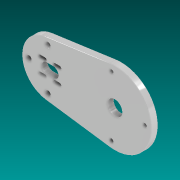
# Autodesk Inventor part: motorplaat
Saved by Autodesk Inventor 2020.2 (Build 242310000, 310)
## iProperties
Created: 2020-05-15
Part Number: motorplaat
Material: Aluminum 6061
Document SubType Name: Modeling
Designer: Svend
Density: 2.7 g/cm^3
Appearance: Aluminum - Polished
Author: Svend
Autodesk Inventor part; units mm, degrees
ref_plane "YZ Plane" through (0, 0, 0) normal (1, 0, 0) x (0, 1, 0)
ref_plane "XZ Plane" through (0, 0, 0) normal (0, 1, 0) x (-1, 0, 0)
ref_plane "XY Plane" through (0, 0, 0) normal (0, 0, 1) x (1, 0, 0)
sketch "Sketch1" plane through (0, 0, 0) normal (0, 0, 1) x (1, 0, 0)
  circle A0 centre (-11.3135, -11.3135) radius 2
  circle A1 centre (-11.3135, 11.3135) radius 2
  circle A2 centre (11.3135, 11.3135) radius 2
  circle A3 centre (11.3135, -11.3135) radius 2
  circle A4 centre (-15.3135, 11.3135) radius 2
  circle A5 centre (-7.3135, 11.3135) radius 2
  circle A6 centre (7.3135, 11.3135) radius 2
  circle A7 centre (15.3135, 11.3135) radius 2
  circle A8 centre (15.3135, -11.3135) radius 2
  circle A9 centre (7.3135, -11.3135) radius 2
  circle A10 centre (-7.3135, -11.3135) radius 2
  circle A11 centre (-15.3135, -11.3135) radius 2
  line L0 (-15.3135, 13.3135) -> (-7.3135, 13.3135)
  line L1 (-7.3135, 9.3135) -> (-15.3135, 9.3135)
  line L2 (-15.3135, -9.3135) -> (-7.3135, -9.3135)
  line L3 (-7.3135, -13.3135) -> (-15.3135, -13.3135)
  line L4 (7.3135, -9.3135) -> (15.3135, -9.3135)
  line L5 (15.3135, -13.3135) -> (7.3135, -13.3135)
  line L6 (15.3135, 9.3135) -> (7.3135, 9.3135)
  line L7 (15.3135, 13.3135) -> (7.3135, 13.3135)
  circle A12 centre (0, 0) radius 8.25
  circle A13 centre (5, 0) radius 8.25
  circle A14 centre (-5, 0) radius 8.25
  line L8 (-5, 8.25) -> (5, 8.25)
  line L9 (5, -8.25) -> (-5, -8.25)
  circle A15 centre (0, 0) radius 42.5
  circle A16 centre (100.143, 0) radius 56.4372
  line L10 (-5.9149, 42.0864) -> (92.2885, 55.888)
  line L11 (-5.9149, -42.0864) -> (92.2885, -55.888)
  line L12 (-13.25, 0) -> (13.25, 0)
  circle A17 centre (100.143, 0) radius 11.5
  arc A18 (-5.9149, 42.0864) -> (-5.9149, -42.0864) centre (0, 0) ccw
  arc A19 (92.2885, -55.888) -> (92.2885, 55.888) centre (100.143, 0) ccw
  line L13 (-42.5, 0) -> (156.5802, 0)
  line L14 (92.2885, 55.888) -> (-5.9149, 42.0864)
  line L15 (-5.9149, -42.0864) -> (92.2885, -55.888)
  line L16 (-3.1314, 22.281) -> (95.0719, 36.0826)
  arc A20 (95.0719, -36.0826) -> (95.0719, 36.0826) centre (100.143, 0) ccw
  line L17 (95.0719, -36.0826) -> (-3.1314, -22.281)
  arc A21 (-3.1314, 22.281) -> (-3.1314, -22.281) centre (0, 0) ccw
  point P0 (146.5802, 0)
  point P1 (95.0719, 46.1809)
  point P2 (95.0719, -46.1809)
  point P3 (-32.5, 0)
  point P4 (-3.1314, 32.3793)
  point P5 (-3.1314, -32.3793)
  dimension "d0" = 4
  dimension "d1" = 22.627
  dimension "d2" = 22.627
  dimension "d3" = 11.3135
  dimension "d4" = 11.3135
  dimension "d5" = 4
  dimension "d6" = 4
  dimension "d7" = 4
  dimension "d8" = 4
  dimension "d9" = 4
  dimension "d10" = 4
  dimension "d11" = 4
  dimension "d12" = 4
  dimension "d15" = 16.5
  dimension "d16" = 5
  dimension "d17" = 5
  dimension "d18" = 85
  dimension "d19" = 8
  dimension "d20" = 100.143
  dimension "d21" = 23
  dimension "d24" = 85
  dimension "d25" = 100.143
  dimension "d26" = 8
  dimension "d27" = 20
  dimension "d28" = 10
  dimension "d29" = 10
  dimension "d30" = 10
  dimension "d31" = 10
  dimension "d32" = 10
  dimension "d33" = 10
  constraints: 36 end point, 36 point on circle, 22 centre point, 15 horizontal alignment, 14 tangent, 13 equal radius, 11 point on line, 6 vertical alignment, 4 coincident, 4 parallel, 3 horizontal, 1 midpoint, 3 other
  measures "d0" diameter of A0
  measures "d1" distance of A1.centre A2.centre
  measures "d2" distance of A3.centre A2.centre
  measures "d3" horizontal distance of point (0, 0) A1.centre
  measures "d4" horizontal distance of point (0, 0) A1.centre
  measures "d5" distance of A2.centre A6.centre
  measures "d6" distance of A7.centre A2.centre
  measures "d7" distance of A3.centre A8.centre
  measures "d8" distance of A9.centre A3.centre
  measures "d9" distance of A0.centre A10.centre
  measures "d10" distance of A11.centre A0.centre
  measures "d11" distance of A1.centre A4.centre
  measures "d12" distance of A5.centre A1.centre
  measures "d15" diameter of A12
  measures "d16" distance of A14.centre A12.centre
  measures "d17" distance of A12.centre A13.centre
  measures "d18" diameter of A15
  measures "d19" angle of L12 L10
  measures "d20" distance of A16.centre point (0, 0)
  measures "d21" diameter of A17
  measures "d24" diameter of A18
  measures "d25" distance of A18.centre A19.centre
  measures "d26" angle of L13 L14
  measures "d27" distance between parallel lines of L14 L16
  measures "d28" distance from line of point (-3.131, -32.379) L17
  measures "d29" distance of L13.end point (146.58, 0)
  measures "d30" distance from line of L16 point (95.072, 46.181)
  measures "d31" distance from line of L16 point (-3.131, 32.379)
  measures "d32" distance from line of point (95.072, -46.181) L17
  measures "d33" distance of L13.start point (-32.5, 0)
extrude "Extrusion1" add sketch "Sketch1" along normal blind 10 contours L13 A15 L17 A21 A14 L9 A13 | A13 L8 A14 L13 A21 L16 A15 | L13 A16 L17 A15 | A15 L16 A16 L13 | L16 A21 L13 A15 | A15 L10 A16 L16 | L17 A16 L11 A15 | A15 L13 A21 L17 | L13 A17 A20 L17 A16 | A16 L16 A20 L13 A17 | A16 L13 A20 L16 | L17 A20 L13 A16
hole "Hole1" at (-3.1314, -32.3793, 0) at (95.0719, -46.1809, 0) at (146.5802, 0, 0) at (95.0719, 46.1809, 0) at (-3.1314, 32.3793, 0) at (-32.5, 0, 0) direction (0, 0, 1) diameter 5.2 depth 10
chamfer "Chamfer1" distance 0.5 angle 45 59 edges at (-42.5, 0, 10) (43.1868, -48.9872, 10) (156.5802, 0, 10) (43.1868, 48.9872, 10) (-42.5, 0, 0) (43.1868, -48.9872, 0) (156.5802, 0, 0) (43.1868, 48.9872, 0) (-5.3135, 11.3135, 10) (-11.3135, 9.3135, 10) (-17.3135, 11.3135, 10) (-11.3135, 13.3135, 10) (-13.25, 0, 10) (0, 8.25, 10) (13.25, 0, 10) (0, -8.25, 10) (-11.3135, -9.3135, 10) (-5.3135, -11.3135, 10) (-11.3135, -13.3135, 10) (-17.3135, -11.3135, 10) (5.3135, 11.3135, 10) (11.3135, 13.3135, 10) (17.3135, 11.3135, 10) (11.3135, 9.3135, 10) (17.3135, -11.3135, 10) (11.3135, -13.3135, 10) (5.3135, -11.3135, 10) (11.3135, -9.3135, 10) (88.643, 0, 0) (88.643, 0, 10) (-5.3135, 11.3135, 0) (-11.3135, 9.3135, 0) (-17.3135, 11.3135, 0) (-11.3135, 13.3135, 0) (-13.25, 0, 0) (0, 8.25, 0) (13.25, 0, 0) (0, -8.25, 0) (-11.3135, -9.3135, 0) (-5.3135, -11.3135, 0) (-11.3135, -13.3135, 0) (-17.3135, -11.3135, 0) (11.3135, 9.3135, 0) (5.3135, 11.3135, 0) (11.3135, 13.3135, 0) (17.3135, 11.3135, 0) (17.3135, -11.3135, 0) (11.3135, -13.3135, 0) (5.3135, -11.3135, 0) (11.3135, -9.3135, 0) (146.5802, -2.6, 0) (95.0719, 43.5809, 0) (95.0719, -48.7809, 0) (-32.5, -2.6, 0) (-3.1314, 29.7793, 0) (-3.1314, -34.9793, 0) (95.0719, -48.7809, 10) (146.5802, -2.6, 10) (95.0719, 43.5809, 10)
chamfer "Chamfer3" distance 2 angle 45 3 edges at (-3.1314, 29.7793, 10) (-32.5, -2.6, 10) (-3.1314, -34.9793, 10)
equation "\"d2\" = d1"
equation "\"d3\" = 0.5 * d2"
equation "\"d4\" = 0.5 * d1"
equation "\"d5\" = d0"
equation "\"d6\" = d5"
equation "\"d7\" = d6"
equation "\"d8\" = d7"
equation "\"d9\" = d5"
equation "\"d10\" = d9"
equation "\"d11\" = d10"
equation "\"d12\" = d11"
equation "\"d17\" = d16"
equation "\"d28\" = 0.5 * d27"
equation "\"d29\" = 0.5 * d27"
equation "\"d30\" = 0.5 * d27"
equation "\"d31\" = 0.5 * d27"
equation "\"d32\" = d30"
equation "\"d33\" = d31"
equation "\"d35\" = d32"
body "Solid1"
